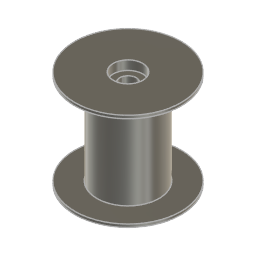
BushingPulley60AIM (Autodesk Fusion 360 design; units mm, degrees)
Autodesk Fusion 360 part; units mm, degrees
note: some values were not read from the file. Set by a fixed rule: which sketch regions a step uses.
sketch "Sketch1" plane through (0, 0, 0) normal (0, 0, 1) x (1, 0, 0)
  circle A0 centre (0, 0) radius 10.2
  line L0 (2.35, -4.25) -> (2.35, -9.45)
  line L1 (-2.35, -4.25) -> (2.35, -4.25)
  line L2 (-2.35, -4.25) -> (2.35, -9.45) construction
  line L3 (2.35, -9.45) -> (-2.35, -9.45)
  line L4 (2.35, -4.25) -> (-2.35, -9.45) construction
  line L5 (-2.35, -9.45) -> (-2.35, -4.25)
  circle A1 centre (0, 0) radius 7.15
  circle A2 centre (0, 0) radius 17.5
  line L6 (0, 0) -> (0, -12)
  point P0 (0, -6.85)
  dimension "d1" = 20.4
  dimension "d2" = 4.7
  dimension "d3" = 5.2
  dimension "d4" = 14.3
  dimension "d5" = 2.9
  dimension "d10" = 35
  constraint coincident A0.centre A1.centre
  constraint horizontal L1
  constraint perpendicular L0 L1
  constraint parallel L1 L3
  constraint parallel L0 L5
  constraint coincident P0 L2
  constraint coincident P0 L4
  constraint perpendicular L3 L6
  constraint coincident P0 L6
  measures "d1" diameter of A0
  measures "d2" distance of L3.end L0.end
  measures "d3" distance of L0.end L0.start
  measures "d4" diameter of A1
  measures "d5" distance of L1 A1
  measures "d10" diameter of A2
extrude "Extrude1" add sketch "Sketch1" along normal blind 31 contours A0 | L0 L1 A1 L6 | L0 L3 A1 L6 | L1 L5 A1 L6 | L3 L5 A1 L6 makes body 1
extrude "Extrude2" add sketch "Sketch1" along normal blind 1 contours A2 bodies 1
extrude "Extrude3" add sketch "Sketch1" along normal blind 1 from surface at 31 separate body contours A0 | L0 L1 A1 L6 | L0 L3 A1 L6 | L1 L5 A1 L6 | L3 L5 A1 L6 | A2 makes body 2
extrude "Extrude4" add sketch "Sketch1" against normal blind 6.5 from surface at 32 separate body contours L0 L1 L5 A1 | L0 L1 A1 L6 | L1 L5 A1 L6 makes body 3
combine "Combine1" operation add target body 2 tool bodies 3
move_face "OffsetFaces1" [suppressed]
sketch "Sketch2" plane through (0, 0, 32) normal (0, 0, 1) x (-1, 0, 0)
  circle A0 centre (0, 0) radius 17.5
  circle A1 centre (0, 0) radius 3
  constraint concentric A0 A1
extrude "Extrude5" cut sketch "Sketch1" against normal blind 5.5 from surface at 31 contours L0 L1 A1 L6 | L1 L5 A1 L6 bodies 1
hole "Hole1" at (0, 0, 32) direction (0, 0, -1) diameter 5.4 depth 15 tip angle 118 counterbore diameter 9.7 counterbore depth 3 bodies 1 2
extrude "Extrude6" cut sketch "Sketch1" along normal blind 8 contours L0 L1 A1 L6 | L1 L5 A1 L6 bodies 1
